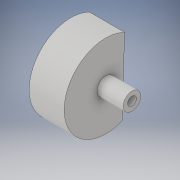
# Autodesk Inventor part: chain stashonary out part
Saved by Autodesk Inventor 2019 (Build 230136000, 136)
## iProperties
Created: 2019-10-22
Part Number: chain stashonary out part
Material: Generic
Document SubType Name: Modeling
Designer: User
Density: 1 g/cm^3
Appearance: Default
Author: User
Autodesk Inventor part; units mm, degrees
ref_plane "YZ Plane" through (0, 0, 0) normal (1, 0, 0) x (0, 1, 0)
ref_plane "XZ Plane" through (0, 0, 0) normal (0, 1, 0) x (-1, 0, 0)
ref_plane "XY Plane" through (0, 0, 0) normal (0, 0, 1) x (1, 0, 0)
sketch "Sketch1" plane through (0, 0, 0) normal (1, 0, 0) x (0, 1, 0)
  circle A0 centre (0, 0) radius 28.575
  circle A1 centre (0, 0) radius 30.1625
  dimension "d0" = 57.15
  dimension "d1" = 60.325
  constraints: 2 centre point, 2 coincident
  measures "d0" diameter of A0
  measures "d1" diameter of A1
extrude "Extrusion1" add sketch "Sketch1" along normal blind 25.4
sketch "Sketch2" plane through (25.4, 0, 0) normal (1, 0, 0) x (0, 0, -1)
  circle A0 centre (0, 0) radius 28.575 projected
  circle A1 centre (0, 0) radius 30.1625 projected
extrude "Extrusion2" add sketch "Sketch2" against normal blind 6.35 contours A0 | A1
sketch "Sketch3" plane through (25.4, 0, 0) normal (1, 0, 0) x (0, 0, -1)
  line L0 (13.6642, 26.8899) -> (11.89, -27.7201)
  circle A0 centre (0, 0) radius 30.1625 projected
  dimension "d6" = 54.61
  constraints: 2 end point, 2 point on circle
  measures "d6" vertical distance of L0.start L0.end
extrude "Extrusion3" cut sketch "Sketch3" against normal through all contours A0 L0 picked at (14.9201, 7.4757)
sketch "Sketch4" plane through (25.4, 0, 0) normal (1, 0, 0) x (0, 0, -1)
  circle A0 centre (0, 0) radius 3.175
  dimension "d9" = 6.35
  constraints: 1 centre point, 1 coincident
  measures "d9" diameter of A0
extrude "Extrusion4" cut sketch "Sketch4" against normal through all
sketch "Sketch5" plane through (25.4, 0, 0) normal (1, 0, 0) x (0, 0, -1)
  circle A0 centre (0, 0) radius 3.175 projected
  circle A1 centre (0, 0) radius 6.35
  dimension "d12" = 6.35
  dimension "d13" = 12.7
  constraints: 1 centre point, 1 coincident
  measures "d12" diameter of A0
  measures "d13" diameter of A1
extrude "Extrusion5" add sketch "Sketch5" along normal blind 19.05
body "Solid1"
